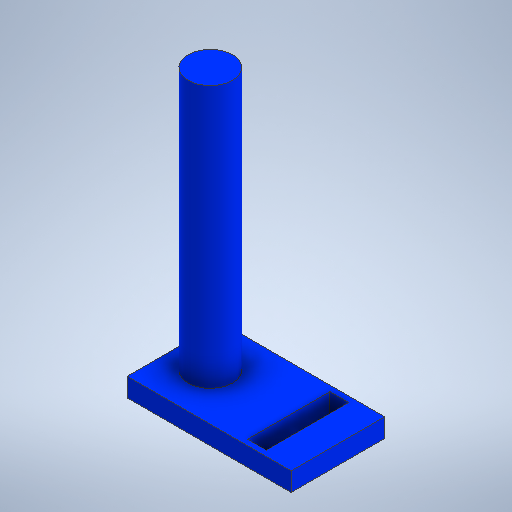
# Autodesk Inventor part: Bluetooth__Base
Saved by Autodesk Inventor 2025.2 (Build 292293000, 293)
## iProperties
Created: 2025-05-04
Part Number: Bluetooth__Base
Material: Generic
Document SubType Name: Modeling
Designer: User
Density: 1 g/cm^3
Appearance: Default
Author: User
Autodesk Inventor part; units mm, degrees
ref_plane "YZ Plane" through (0, 0, 0) normal (1, 0, 0) x (0, 1, 0)
ref_plane "XZ Plane" through (0, 0, 0) normal (0, 1, 0) x (-1, 0, 0)
ref_plane "XY Plane" through (0, 0, 0) normal (0, 0, 1) x (1, 0, 0)
sketch "Sketch1" plane through (0, 0, 0) normal (0, 1, 0) x (-1, 0, 0)
  circle A0 centre (0, 0) radius 4.75
  line L0 (7.75, 0) -> (7.75, -10)
  line L1 (7.75, -10) -> (-27.25, -10)
  line L2 (-27.25, -10) -> (-27.25, 10)
  line L3 (-27.25, 10) -> (7.75, 10)
  line L4 (7.75, 10) -> (7.75, 0)
  line L5 (-4.75, 0) -> (-16.75, 0)
  line L6 (-16.75, -10) -> (-16.75, -8.8)
  line L7 (-16.75, 10) -> (-16.75, 8.8)
  line L8 (-16.75, 8.8) -> (-16.75, -8.8)
  line L9 (-16.75, -8.8) -> (-20.75, -8.8)
  line L10 (-20.75, -8.8) -> (-20.75, 8.8)
  line L11 (-20.75, 8.8) -> (-16.75, 8.8)
  line L12 (-20.75, -8.8) -> (-20.75, -10)
  line L13 (-20.75, 8.8) -> (-20.75, 10)
  dimension "d0" = 9.5
  dimension "d2" = 10
  dimension "d3" = 35
  dimension "d4" = 20
  dimension "d5" = 12
  dimension "d6" = 1.2
  dimension "d7" = 1.2
  dimension "d8" = 4
  constraints: 28 end point, 6 perpendicular, 6 point on line, 2 collinear, 2 horizontal, 2 vertical, 1 coincident, 1 horizontal alignment, 2 other
  measures "d2" distance of L0.start L0.end
  measures "d3" distance of L0.end L1.end
  measures "d4" distance of L1.end L2.end
  measures "d5" distance of L5.start L5.end
  measures "d6" distance of L6.start L6.end
  measures "d7" distance of L7.start L7.end
  measures "d8" distance of L6.end L9.end
extrude "Extrusion1" add sketch "Sketch1" along normal blind 60 contours A0
extrude "Extrusion2" add sketch "Sketch1" along normal blind 4 contours L8 L7 L3 L4 L0 L1 L6
extrude "Extrusion3" add sketch "Sketch1" along normal blind 4 contours L6 L1 L12 L9
extrude "Extrusion4" add sketch "Sketch1" along normal blind 4 contours L11 L13 L3 L7
extrude "Extrusion5" add sketch "Sketch1" along normal blind 4 contours L10 L12 L1 L2 L3 L13
body "Solid1"
